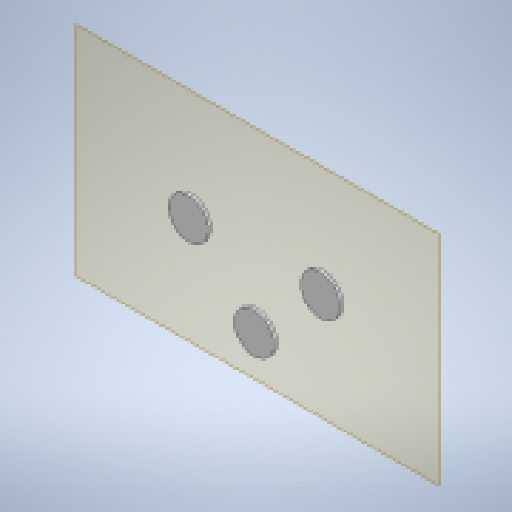
# Autodesk Inventor part: Zaślepki
Saved by Autodesk Inventor 2025.2 (Build 292293000, 293)
## iProperties
Created: 2025-03-23
Part Number: Zaślepki
Material: PC/ABS Plastic
Document SubType Name: Modeling
Designer: danie
Density: 1.1 g/cm^3
Appearance: Smooth - White
Author: danie
Autodesk Inventor part; units mm, degrees
ref_plane "YZ Plane" through (0, 0, 0) normal (1, 0, 0) x (0, 1, 0)
ref_plane "XZ Plane" through (0, 0, 0) normal (0, 1, 0) x (-1, 0, 0)
ref_plane "XY Plane" through (0, 0, 0) normal (0, 0, 1) x (1, 0, 0)
ref_plane "Work Plane1" through (-71.5489, -58.6984, 0) normal (0, 0, 1) x (1, 0, 0)
sketch "Sketch1" plane through (-71.5489, -58.6984, 0) normal (0, 0, 1) x (1, 0, 0)
  line L0 (759.116, -466.2748) -> (759.116, 295.7252) projected
  line L1 (759.116, 295.7252) -> (-510.884, 295.7252) projected
  line L2 (-510.884, 295.7252) -> (-510.884, -466.2748) projected
  line L3 (-510.884, -466.2748) -> (759.116, -466.2748) projected
  arc A0 (453.0245, -72.0929) -> (303.2076, -72.0929) centre (378.116, -86.0629) ccw projected
  arc A1 (198.2364, -325.3048) -> (48.4195, -325.3048) centre (123.3279, -339.2748) ccw projected
  arc A2 (453.0245, -72.0929) -> (303.2076, -72.0929) centre (378.116, -86.0629) ccw projected
  arc A3 (198.2364, -325.3048) -> (48.4195, -325.3048) centre (123.3279, -339.2748) ccw projected
  arc A4 (-204.7924, -98.4567) -> (-54.9755, -98.4567) centre (-129.884, -84.4867) ccw projected
  line L4 (276.516, -72.0929) -> (303.2076, -72.0929) projected
  line L5 (453.0245, -72.0929) -> (479.716, -72.0929) projected
  line L6 (479.716, -72.0929) -> (479.716, -100.0329) projected
  line L7 (479.716, -100.0329) -> (453.0245, -100.0329) projected
  arc A5 (303.2076, -100.0329) -> (453.0245, -100.0329) centre (378.116, -86.0629) ccw projected
  line L8 (303.2076, -100.0329) -> (276.516, -100.0329) projected
  line L9 (276.516, -100.0329) -> (276.516, -72.0929) projected
  line L10 (21.7279, -325.3048) -> (48.4195, -325.3048) projected
  line L11 (198.2364, -325.3048) -> (224.9279, -325.3048) projected
  line L12 (224.9279, -325.3048) -> (224.9279, -353.2448) projected
  line L13 (224.9279, -353.2448) -> (198.2364, -353.2448) projected
  arc A6 (48.4195, -353.2448) -> (198.2364, -353.2448) centre (123.3279, -339.2748) ccw projected
  line L14 (48.4195, -353.2448) -> (21.7279, -353.2448) projected
  line L15 (21.7279, -353.2448) -> (21.7279, -325.3048) projected
  line L16 (-28.284, -98.4567) -> (-54.9755, -98.4567) projected
  line L17 (-204.7924, -98.4567) -> (-231.484, -98.4567) projected
  line L18 (-231.484, -98.4567) -> (-231.484, -70.5167) projected
  line L19 (-231.484, -70.5167) -> (-204.7924, -70.5167) projected
  arc A7 (-54.9755, -70.5167) -> (-204.7924, -70.5167) centre (-129.884, -84.4867) ccw projected
  line L20 (-54.9755, -70.5167) -> (-28.284, -70.5167) projected
  line L21 (-28.284, -70.5167) -> (-28.284, -98.4567) projected
  arc A8 (-204.7924, -98.4567) -> (-54.9755, -98.4567) centre (-129.884, -84.4867) ccw projected
  line L22 (174.1279, -135.2867) -> (72.5279, -135.2867) projected
  line L23 (72.5279, -135.2867) -> (72.5279, -33.6867) projected
  line L24 (72.5279, -33.6867) -> (174.1279, -33.6867) projected
  line L25 (174.1279, -33.6867) -> (174.1279, -135.2867) projected
  line L26 (174.1279, 149.6752) -> (174.1279, 238.5752) projected
  line L27 (174.1279, 238.5752) -> (428.1279, 238.5752) projected
  line L28 (428.1279, 238.5752) -> (428.1279, 149.6752) projected
  line L29 (428.1279, 149.6752) -> (174.1279, 149.6752) projected
  line L30 (72.5279, 149.6752) -> (-181.4721, 149.6752) projected
  line L31 (-181.4721, 149.6752) -> (-181.4721, 238.5752) projected
  line L32 (-181.4721, 238.5752) -> (72.5279, 238.5752) projected
  line L33 (72.5279, 238.5752) -> (72.5279, 149.6752) projected
  point P0 (71.5489, 58.6984)
  point P1 (325.793, 63.2483)
  point P2 (71.0049, -189.9636)
  point P3 (-182.207, 64.8245)
extrude "Extrusion1" add sketch "Sketch1" along normal blind 12.7 contours L5 L6 L7 A5 L8 L9 L4 A0 | L11 L12 L13 A6 L14 L15 L10 A1 | L17 L18 L19 A7 L20 L21 L16 A4
body "Solid1"
